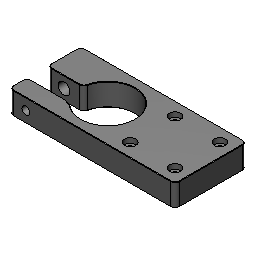
Nikon10x_objective_holder (Autodesk Fusion 360 design; units mm, degrees)
Autodesk Fusion 360 part; units mm, degrees
sketch "Base profile and screw holes" plane through (0, 0, 0) normal (0, 0, 1) x (1, 0, 0)
  line L0 (15, 15) -> (-15, 15)
  line L1 (-15, 15) -> (-15, -17)
  line L2 (-15, -17) -> (15, -17)
  line L3 (15, -17) -> (15, 15)
  circle A0 centre (-11, -11) radius 1.25
  circle A1 centre (9, -11) radius 1.25
  circle A2 centre (-11, 9) radius 1.25
  circle A3 centre (9, 9) radius 1.25
  dimension "d1" = 30
  dimension "d5" = 4
  dimension "d8" = 20
  dimension "d9" = 2.5
  dimension "d10" = 20
  dimension "d40" = 11
  dimension "d41" = 6
  dimension "d42" = 6
  constraint horizontal L0
  constraint perpendicular L0 L1
  constraint parallel L0 L2
  constraint parallel L1 L3
  constraint horizontal A0.centre A1.centre
  constraint vertical A0.centre A2.centre
  constraint vertical A1.centre A3.centre
  constraint horizontal A2.centre A3.centre
  constraint equal A2 A3
  constraint equal A0 A2
  constraint equal A1 A2
  measures "d1" distance of L0.start L0.end
  measures "d5" distance of L1 A0.centre
  measures "d8" distance of A0.centre A1.centre
  measures "d9" diameter of A2
  measures "d10" distance of A0.centre A2.centre
  measures "d40" vertical distance of origin A0.centre
  measures "d41" distance of L2 A0.centre
  measures "d42" distance of L0 A2.centre
extrude "Extrude1" add sketch "Base profile and screw holes" along normal blind 10 makes body 1
ref_plane "WorkPlane1" through (0, 0, -30) normal (0, 0, 1) x (1, 0, 0)
sketch "Original holder" plane through (0, 0, -30) normal (0, 0, 1) x (1, 0, 0)
  circle A0 centre (-31, 0) radius 12.75
  circle A1 centre (-11, -11) radius 1.25
  line L0 (-14.1024, 16) -> (-47.8976, 16)
  line L1 (-47.8976, 16) -> (-47.8976, -16)
  line L2 (-47.8976, -16) -> (-14.1024, -16)
  line L3 (-14.1024, -16) -> (-14.1024, 16)
  line L4 (-14.1024, 16) -> (-47.8976, -16) construction
  line L5 (-47.8976, 16) -> (-14.1024, -16) construction
  line L6 (-15, 15) -> (-15, -17)
  point P0 (-31, 0)
  dimension "d16" = 25.5
  dimension "d17" = 20
  constraint horizontal origin A0.centre
  constraint horizontal L0
  constraint perpendicular L0 L1
  constraint parallel L0 L2
  constraint parallel L1 L3
  constraint coincident L4 P0
  constraint coincident L5 P0
  constraint coincident P0 A0.centre
  constraint equal L3 L6
  measures "d16" diameter of A0
  measures "d17" horizontal distance of P0 A1.centre
extrude "Extrude2" add sketch "Original holder" against normal blind 5 separate body contours L0 L1 L2 L3 makes body 2
sketch "Nikon 10x objective" plane through (0, 0, 0) normal (0, 1, 0) x (1, 0, 0)
  line L0 (-43.4233, 29.7385) -> (-30.9233, 29.7385)
  line L1 (-30.9233, 29.7385) -> (-30.9233, 34.7385)
  line L2 (-30.9233, 34.7385) -> (-43.4233, 34.7385)
  line L3 (-43.4233, 34.7385) -> (-43.4233, 29.7385)
  line L4 (-30.9233, 29.7385) -> (-44.9233, 29.7385)
  line L5 (-44.9233, 29.7385) -> (-44.9233, 24.7385)
  line L6 (-44.9233, 24.7385) -> (-30.9233, 24.7385)
  line L7 (-30.9233, 24.7385) -> (-30.9233, 29.7385)
  line L8 (-44.9233, 24.7385) -> (-42.9233, 22.7376)
  line L9 (-44.9233, 24.7385) -> (-39.0718, 24.7385) construction
  line L10 (-30.9233, 24.7385) -> (-42.9233, 24.7385)
  line L11 (-42.9233, 24.7385) -> (-42.9233, -13.2615)
  line L12 (-42.9233, -13.2615) -> (-30.9233, -13.2615)
  line L13 (-30.9233, -13.2615) -> (-30.9233, 24.7385)
  line L14 (-30.9233, -13.2615) -> (-40.1733, -13.2615)
  line L15 (-40.1733, -13.2615) -> (-40.1733, -16.7692)
  line L16 (-30.9233, -17.6525) -> (-30.9233, -13.2615)
  line L17 (-40.1733, -16.7692) -> (-34.1733, -27.1615)
  line L18 (-30.9233, -17.6525) -> (-30.9233, -27.1615)
  line L19 (-34.1733, -27.1615) -> (-30.9233, -27.1615)
  line L20 (-42.9233, -10.9477) -> (-41.5874, -13.2615)
  line L21 (-42.9233, -10.9477) -> (-41.0507, -10.9477) construction
  dimension "d20" = 12.5
  dimension "d21" = 5
  dimension "d22" = 14
  dimension "d23" = 5
  dimension "d26" = 12
  dimension "d29" = 9.25
  dimension "d31" = 3.25
  dimension "d33" = 43
  dimension "d34" = 60
  dimension "d35" = 13.9
  dimension "d36" = 60
  constraint horizontal L0
  constraint vertical L1
  constraint horizontal L2
  constraint vertical L3
  constraint horizontal L4
  constraint vertical L5
  constraint horizontal L6
  constraint vertical L7
  constraint horizontal L9
  constraint horizontal L10
  constraint vertical L11
  constraint horizontal L12
  constraint vertical L13
  constraint coincident L8.end L11
  constraint horizontal L14
  constraint vertical L15
  constraint vertical L16
  constraint coincident L18 L19.end
  constraint perpendicular L18 L19
  constraint horizontal L21
  constraint coincident L11 L20.start
  constraint coincident L12 L20.end
  measures "d20" distance of L0.start L0.end
  measures "d21" distance of L0.start L2.end
  measures "d22" distance of L0.end L4.end
  measures "d23" distance of L4.end L5.end
  measures "d26" distance of L6.end L10.end
  measures "d29" distance of L12.end L14.end
  measures "d31" distance of L17.end L18.end
  measures "d33" vertical distance of L4.end L11.end
  measures "d34" angle of L20 L21
  measures "d35" distance of L14 L19
  measures "d36" angle of L12 L17
revolve "Revolve1" add sketch "Nikon 10x objective" angle 360 about axis through (-30.9233, 0, 13.2615) along (0, 0, -1) separate body contours L0 L1 L2 L3 L4 | L0 L4 L5 L6 L7 L10 | L6 L10 L11 L12 L13 L14 L20 | L6 L8 L11 | L12 L14 L15 L16 L17 L18 L19 makes body 3
sketch "Main body of holder" plane through (0, 0, 0) normal (0, 0, 1) x (1, 0, 0)
  circle A0 centre (-31, -1) radius 12
  line L0 (-11, 9) -> (-11, -11) construction
  line L1 (-15, 15) -> (-59, 15)
  line L2 (-59, 15) -> (-59, -17)
  line L3 (-59, -17) -> (-15, -17)
  line L4 (-15, -17) -> (-15, 15)
  line L5 (-59, -9) -> (-39.9443, -9)
  line L6 (-59, 0) -> (-42.9583, 0)
  point P0 (-11, -11)
  point P1 (-11, 9)
  point P2 (-11, -1)
  point P3 (-15, 15)
  point P4 (-15, -17)
  dimension "d38" = 24
  dimension "d39" = 20
  dimension "d43" = 15
  dimension "d44" = 8
  dimension "d45" = 44
  constraint coincident P1 L0.start
  constraint coincident P0 L0.end
  constraint midpoint L0 P2
  constraint horizontal A0.centre P2
  constraint horizontal L1
  constraint vertical L2
  constraint horizontal L3
  constraint vertical L4
  constraint coincident P3 L1.start
  constraint coincident P4 L3.end
  constraint coincident L2 L5.start
  constraint coincident A0 L5.end
  constraint perpendicular L2 L5
  constraint coincident L2 L6.start
  constraint coincident A0 L6.end
  constraint perpendicular L2 L6
  measures "d38" diameter of A0
  measures "d39" horizontal distance of A0.centre P0
  measures "d43" distance of L1 L6
  measures "d44" distance of L3 L5
  measures "d45" distance of P3 L1.end
extrude "Extrude3" add sketch "Main body of holder" along normal up to surface (10 mm away) contours A0 L1 L2 L3 L4 L5 L6 bodies 1
sketch "Hole for bolt that goes into heat-set insert" plane through (0, -17, 0) normal (0, -1, 0) x (1, 0, 0)
  line L0 (-59, 0) -> (15, 0)
  line L1 (15, 0) -> (15, 10)
  line L2 (15, 10) -> (-59, 10)
  line L3 (-59, 10) -> (-59, 0)
  circle A0 centre (-51.5415, 5) radius 1.75
  point P0 (-59, 5)
  dimension "d48" = 3.5
  constraint midpoint L3 P0
  constraint horizontal A0.centre P0
  measures "d48" diameter of A0
extrude "Extrude4" cut sketch "Hole for bolt that goes into heat-set insert" against normal up to surface (8 mm away) contours A0 bodies 1
chamfer "Chamfer1" distance 2 angle 45 1 edges at (-39.9443, -9, 5) on bodies 1
sketch "Hole for heat-set insert" plane through (0, 15, 0) normal (0, 1, 0) x (-1, 0, 0)
  line L0 (-15, 0) -> (59, 0)
  line L1 (59, 0) -> (59, 10)
  line L2 (59, 10) -> (-15, 10)
  line L3 (-15, 10) -> (-15, 0)
  circle A0 centre (51.5415, 5) radius 2.6
  circle A1 centre (51.5415, 5) radius 1.75
  dimension "d52" = 5.2
  constraint concentric A0 A1
  measures "d52" diameter of A0
extrude "Extrude5" cut sketch "Hole for heat-set insert" against normal up to surface (15 mm away) contours A0 | A1 bodies 1
fillet "Fillet3" radius 2 7 edges at (-59, 15, 5) (-59, 0, 5) (-59, -9, 5) (-59, -17, 5) (-42.9583, 0, 5) (15, -17, 5) (15, 15, 5) on bodies 1
chamfer "Chamfer2" distance 0.2 angle 45 34 edges at (-22, 15, 10) (14.4142, 14.4142, 10) (15, -1, 10) (14.4142, -16.4142, 10) (-22, -17, 10) (-58.4142, -16.4142, 10) (-59, -13, 10) (-58.4142, -9.5858, 10) (-49.4721, -9, 10) (-19.6882, 3.0054, 10) (-43.4212, 0.4416, 10) (-50.8374, 0, 10) (-58.4142, 0.5858, 10) (-59, 7.5, 10) (-58.4142, 14.4142, 10) (-22, 15, 0) (14.4142, 14.4142, 0) (15, -1, 0) (14.4142, -16.4142, 0) (-22, -17, 0) (-58.4142, -16.4142, 0) (-59, -13, 0) (-58.4142, -9.5858, 0) (-49.4721, -9, 0) (-19.6882, 3.0054, 0) (-43.4212, 0.4416, 0) (-50.8374, 0, 0) (-58.4142, 0.5858, 0) (-59, 7.5, 0) (-58.4142, 14.4142, 0) (-12.1654, -10.548, 0) (-12.1654, 9.452, 0) (7.8346, 9.452, 0) (7.8346, -10.548, 0) on bodies 1
chamfer "Chamfer2" distance 0.2 angle 45 2 edges at (-40.2178, -9.6872, 0) (-40.2178, -9.6872, 10) on bodies 1
sketch "Counterbore for bolts that attach to microscope stage" plane through (0, 0, 10) normal (0, 0, 1) x (-1, 0, 0)
  circle A0 centre (11, -9) radius 2.5
  circle A1 centre (-9, -9) radius 2.5
  circle A2 centre (11, 11) radius 2.5
  circle A3 centre (-9, 11) radius 2.5
  point P0 (11, -9)
  point P1 (-9, -9)
  point P2 (-9, 11)
  point P3 (11, 11)
  dimension "d62" = 5
  constraint coincident P0 A0.centre
  constraint equal A0 A1
  constraint equal A0 A2
  constraint equal A0 A3
  constraint coincident P1 A1.centre
  constraint coincident P2 A3.centre
  constraint coincident P3 A2.centre
  measures "d62" diameter of A0
extrude "Extrude6" cut sketch "Counterbore for bolts that attach to microscope stage" against normal blind 2.2 bodies 1
sketch "Counterbore for bolt that goes into the heat-set insert" plane through (0, 15, 0) normal (0, -1, 0) x (1, 0, 0)
  circle A0 centre (-51.5415, 5) radius 3.3
  point P0 (-51.5415, 5)
  dimension "d65" = 6.6
  constraint coincident P0 A0.centre
  measures "d65" diameter of A0
extrude "Extrude8" cut sketch "Counterbore for bolt that goes into the heat-set insert" along normal blind 7 bodies 1
hidden bodies 2 3
named bodies: "Holder for Nikon 10x objective", "Original objective holder template", "Nikon10x objective"
